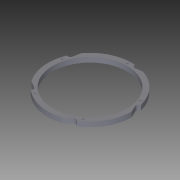
# Autodesk Inventor part: innerring
Saved by Autodesk Inventor 2015 (Build 190159000, 159)
## iProperties
Created: 2015-03-04
Part Number: innerring
Material: Generic
Document SubType Name: Modeling
Designer: janov_000
Density: 1 g/cm^3
Appearance: Default
Author: janov_000
Autodesk Inventor part; units mm, degrees
ref_plane "YZ Plane" through (0, 0, 0) normal (1, 0, 0) x (0, 1, 0)
ref_plane "XZ Plane" through (0, 0, 0) normal (0, 1, 0) x (-1, 0, 0)
ref_plane "XY Plane" through (0, 0, 0) normal (0, 0, 1) x (1, 0, 0)
sketch "Sketch1" plane through (0, 0, 0) normal (0, 0, 1) x (1, 0, 0)
  circle A0 centre (77.3169, -37.9173) radius 75
  circle A1 centre (77.3169, -37.9173) radius 85
  circle A2 centre (77.3169, -37.9173) radius 75 projected
  point P0 (0, 0)
  dimension "d0" = 150
  dimension "d1" = 170
  constraints: 2 centre point, 2 coincident
  measures "d0" diameter of A0
  measures "d1" diameter of A1
extrude "Extrusion1" add sketch "Sketch1" along normal blind 10
sketch "Sketch3" plane through (77.3169, -37.9173, 10) normal (0, 0, 1) x (1, 0, 0)
  circle A0 centre (-76.5194, 37.0443) radius 2.5 construction
  circle A1 centre (-58.877, -61.3269) radius 2.5 construction
  circle A2 centre (40.1314, -74.9464) radius 2.5 construction
  circle A3 centre (83.6796, 15.0075) radius 2.5 construction
  circle A4 centre (11.5854, 84.2216) radius 2.5 construction
  line L0 (40.1314, -74.9464) -> (25.5443, -88.6291) construction
  line L1 (36.3686, -70.935) -> (21.7815, -84.6177)
  line L2 (29.307, -92.6406) -> (43.8941, -78.9579)
  arc A5 (43.8941, -78.9579) -> (36.3686, -70.935) centre (40.1314, -74.9464) ccw
  arc A6 (21.7815, -84.6177) -> (29.307, -92.6406) centre (25.5443, -88.6291) ccw
  line L3 (40.1314, -74.9464) -> (48.951, -91.4173) construction
  circle A7 centre (0, 0) radius 85 construction
  line L4 (78.7017, 12.6685) -> (87.207, -5.4328)
  line L5 (97.1628, -0.7549) -> (88.6574, 17.3465)
  arc A8 (88.6574, 17.3465) -> (78.7017, 12.6685) centre (83.6796, 15.0075) ccw
  arc A9 (87.207, -5.4328) -> (97.1628, -0.7549) centre (92.1849, -3.0939) ccw
  line L6 (12.2717, 78.7645) -> (32.1154, 81.26)
  line L7 (30.7429, 92.174) -> (10.8992, 89.6786)
  arc A10 (10.8992, 89.6786) -> (12.2717, 78.7645) centre (11.5854, 84.2216) ccw
  arc A11 (32.1154, 81.26) -> (30.7429, 92.174) centre (31.4292, 86.717) ccw
  line L8 (-71.1174, 36.0107) -> (-67.3586, 55.6543)
  line L9 (-78.1626, 57.7216) -> (-81.9214, 38.078)
  arc A12 (-81.9214, 38.078) -> (-71.1174, 36.0107) centre (-76.5194, 37.0443) ccw
  arc A13 (-67.3586, 55.6543) -> (-78.1626, 57.7216) centre (-72.7606, 56.6879) ccw
  line L10 (-56.2246, -56.5087) -> (-73.7453, -46.8638)
  line L11 (-79.0501, -56.5001) -> (-61.5294, -66.1451)
  arc A14 (-61.5294, -66.1451) -> (-56.2246, -56.5087) centre (-58.877, -61.3269) ccw
  arc A15 (-73.7453, -46.8638) -> (-79.0501, -56.5001) centre (-76.3977, -51.6819) ccw
  point P0 (-77.3169, 37.9173)
  point P1 (32.8378, -81.7878)
  dimension "d22" = 11
  dimension "d23" = 75
  dimension "d24" = 20
  dimension "d27" = 360
  constraints: 26 end point, 20 point on circle, 10 centre point, 4 tangent, 1 coincident, 1 line through centre, 1 midpoint, 1 parallel, 51 other
  measures "d22" diameter of A6
  measures "d23" angle of L0 L3
  measures "d24" distance of L0.start L0.end
extrude "Extrusion5" cut sketch "Sketch3" against normal blind 10
sketch "Sketch4" plane through (0, 0, 10) normal (0, 0, 1) x (1, 0, 0)
  circle A0 centre (0.3478, -16.1054) radius 2.5 projected
  circle A1 centre (32.7878, -104.379) radius 2.5 projected
  circle A2 centre (126.7655, -100.8047) radius 2.5 projected
  circle A3 centre (152.4069, -10.3221) radius 2.5 projected
  circle A4 centre (74.2765, 42.0249) radius 2.5 projected
  point P0 (0, 0)
  constraints: 5 coincident
hole "Hole1" at (32.7878, -104.379, 10) at (126.7655, -100.8047, 10) at (152.4069, -10.3221, 10) at (74.2765, 42.0249, 10) at (0.3478, -16.1054, 10) direction (0, 0, -1) diameter 5 end through all
body "Solid1"
